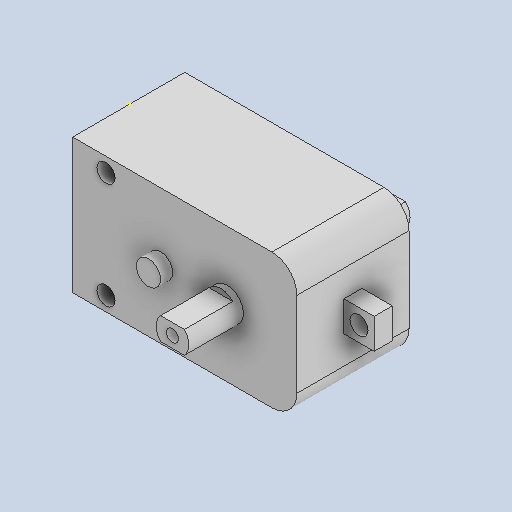
# Autodesk Inventor part: TT motor output
Saved by Autodesk Inventor 2022 (Build 260153070, 153G)
## iProperties
Created: 2021-11-27
Part Number: TT motor output
Material: Generic
Document SubType Name: Modeling
Designer: a laptop
Density: 1 g/cm^3
Appearance: Default
Author: a laptop
Autodesk Inventor part; units mm, degrees
ref_plane "YZ Plane" through (0, 0, 0) normal (1, 0, 0) x (0, 1, 0)
ref_plane "XZ Plane" through (0, 0, 0) normal (0, 1, 0) x (-1, 0, 0)
ref_plane "XY Plane" through (0, 0, 0) normal (0, 0, 1) x (1, 0, 0)
sketch "Sketch1" plane through (0, 0, 0) normal (0, 0, 1) x (1, 0, 0)
  line L0 (0, 0) -> (32.875, 0)
  line L1 (37, 0) -> (37, -4.125)
  line L2 (37, -22.25) -> (0, -22.25)
  line L3 (0, -22.25) -> (0, -11.125)
  line L4 (0, -11.125) -> (37, -11.125) construction
  line L5 (0, -11.125) -> (0, 0)
  circle A0 centre (14.5, -11.125) radius 2
  circle A1 centre (5.5, -2.375) radius 1.5
  arc A2 (37, -4.125) -> (32.875, 0) centre (32.875, -4.125) ccw
  line L6 (32.875, 0) -> (37, 0)
  line L7 (37, -4.125) -> (37, -22.25)
  arc A3 (32.875, -22.25) -> (37, -18.125) centre (32.875, -18.125) ccw
  circle A4 centre (5.5, -19.875) radius 1.5
  circle A5 centre (25.47, -11.125) radius 2.7
  line L8 (23.5034, -9.275) -> (27.4366, -9.275)
  line L9 (27.4366, -12.975) -> (23.5034, -12.975)
  point P0 (36.5, -18.125)
  point P1 (36.9, -18.125)
  dimension "d6" = 4
  dimension "d8" = 3
  dimension "d11" = 5.5
  dimension "d12" = 22.25
  dimension "d13" = 8.75
  dimension "d16" = 14.5
  dimension "d17" = 14
  dimension "d18" = 37
  dimension "d19" = 3.7
  dimension "d28" = 5.4
  dimension "d29" = 11.53
  constraints: 20 end point, 9 point on circle, 7 parallel, 6 centre point, 6 perpendicular, 6 point on line, 4 symmetric about line, 3 equal length, 3 horizontal, 2 tangent, 1 coincident, 1 horizontal alignment, 1 vertical alignment, 2 other
  measures "d6" diameter of A0
  measures "d8" diameter of A1
  measures "d11" distance from line of L5 A1.centre
  measures "d12" distance of L1.start L2.start
  measures "d13" distance from line of L4 A1.centre
  measures "d16" distance from line of L3 A0.centre
  measures "d17" distance of A3.end A2.start
  measures "d18" distance of L0.start L1.start
  measures "d19" distance between parallel lines of L9 L8
  measures "d28" diameter of A5
  measures "d29" distance from line of L7 A5.centre
extrude "Extrusion1" add sketch "Sketch1" along normal mid plane 18.5 contours L0 A2 L7 A3 L2 L3 L5
extrude "Extrusion2" add sketch "Sketch1" along normal mid plane 22.5 contours A0
extrude "Extrusion3" add sketch "Sketch1" along normal mid plane 20.5 contours A5 L9 L8 | L8 A5 | A5 L9
extrude "Extrusion4" add sketch "Sketch1" along normal mid plane 36.5 contours A5 L9 L8
sketch "Sketch2" plane through (0, -22.25, 9.25) normal (-1, 0, 0) x (0, 0, 1)
  point P0 (-9.25, 22.25)
sketch "Sketch3" plane through (0, 0, -18.25) normal (0, 0, -1) x (-1, 0, 0)
  circle A0 centre (-25.47, -11.125) radius 1
  arc A1 (-23.5034, -12.975) -> (-23.5034, -9.275) centre (-25.47, -11.125) ccw projected
  point P0 (0, 0)
  dimension "d30" = 2
  constraints: 1 centre point, 1 concentric
  measures "d30" diameter of A0
extrude "Extrusion5" cut sketch "Sketch3" against normal blind 5
sketch "Sketch4" plane through (0, 0, 18.25) normal (0, 0, 1) x (1, 0, 0)
  circle A0 centre (25.47, -11.125) radius 1
  arc A1 (27.4366, -12.975) -> (27.4366, -9.275) centre (25.47, -11.125) ccw projected
  point P0 (0, 0)
  dimension "d33" = 2
  constraints: 1 centre point, 1 concentric
  measures "d33" diameter of A0
extrude "Extrusion6" cut sketch "Sketch4" against normal blind 5
sketch "Sketch5" plane through (37, -18.125, 9.25) normal (1, 0, 0) x (0, 0, -1)
  line L0 (9.25, 18.125) -> (9.25, 0) construction
  line L1 (18.5, 0) -> (0, 0) projected
  line L2 (7.75, 9.625) -> (10.75, 9.625)
  line L3 (10.75, 9.625) -> (10.75, 4.625)
  line L4 (10.75, 4.625) -> (9.25, 4.625)
  line L5 (7.75, 4.625) -> (7.75, 9.625)
  line L6 (9.25, 4.625) -> (7.75, 4.625)
  dimension "d36" = 3
  dimension "d37" = 5
  dimension "d38" = 8.5
  constraints: 12 end point, 3 parallel, 1 coincident, 1 collinear, 1 horizontal, 1 midpoint, 1 perpendicular, 1 point on line, 1 vertical
  measures "d36" distance of L2.start L2.end
  measures "d37" distance of L2.end L3.end
  measures "d38" distance from line of point (9.25, 18.125) L2
extrude "Extrusion7" add sketch "Sketch5" along normal blind 5
sketch "Sketch6" plane through (37, -13.5, 1.5) normal (0, 0, 1) x (1, 0, 0)
  circle A0 centre (2.5, 2.5) radius 1.5
  line L0 (5, 0) -> (5, 2.5) construction
  line L1 (5, 5) -> (5, 0) construction
  line L2 (5, 0) -> (5, 5) construction
  line L3 (5, 2.5) -> (0, 2.5) construction
  line L4 (5, 2.5) -> (5, 5) construction
  line L5 (5, 5) -> (5, 0) construction
  line L6 (0, 5) -> (5, 5) construction
  line L7 (2.5, 5) -> (2.5, 0) construction
  line L8 (0, 0) -> (5, 0) projected
  line L9 (0, 5) -> (0, 0) construction
  line L10 (0, 5) -> (0, 2.5) construction
  point P0 (-37, 13.5)
  point P1 (2.5, 2.5)
  dimension "d41" = 3
  constraints: 12 end point, 4 midpoint, 2 collinear, 1 centre point, 1 coincident, 1 horizontal, 1 vertical
  measures "d41" diameter of A0
extrude "Extrusion8" cut sketch "Sketch6" against normal blind 5
ref_plane "Work Plane1" through (0, 0, 0) normal (0, 0, 1) x (1, 0, 0)
ref_plane "Work Plane2" through (0, -11.125, 9.25) normal (0, -1, 0) x (1, 0, 0)
body "Solid1"
